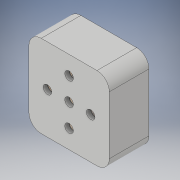
# Autodesk Inventor part: bottom
Saved by Autodesk Inventor 2019 (Build 230136000, 136)
## iProperties
Created: 2019-08-20
Part Number: bottom
Material: Generic
Document SubType Name: Modeling
Designer: assman
Density: 1 g/cm^3
Appearance: Default
Author: assman
## iProperties of the stored document bottom_3DPrint.ipt
Created: 2019-08-20
Part Number: bottom_3DPrint
Material: Generic
Document SubType Name: Modeling
Designer: assman
Density: 1 g/cm^3
Appearance: Default
Author: assman
Autodesk Inventor part; units mm, degrees
ref_plane "YZ Plane" through (0, 0, 0) normal (1, 0, 0) x (0, 1, 0)
ref_plane "XZ Plane" through (0, 0, 0) normal (0, 1, 0) x (-1, 0, 0)
ref_plane "XY Plane" through (0, 0, 0) normal (0, 0, 1) x (1, 0, 0)
ref_plane "Work Plane1" through (0, 0, 0) normal (0, 0, 1) x (-1, 0, 0)
sketch "Sketch1" plane through (0, 0, 0) normal (0, 0, 1) x (-1, 0, 0)
  line L0 (-17.4798, 9.425) -> (-17.4798, -9.425)
  arc A0 (-17.4798, -9.425) -> (-13.4798, -13.425) centre (-13.4798, -9.425) ccw
  line L1 (-13.4798, -13.425) -> (4.6702, -13.425)
  arc A1 (4.6702, -13.425) -> (8.6702, -9.425) centre (4.6702, -9.425) ccw
  line L2 (8.6702, -9.425) -> (8.6702, 9.425)
  arc A2 (8.6702, 9.425) -> (4.6702, 13.425) centre (4.6702, 9.425) ccw
  line L3 (4.6702, 13.425) -> (-0.4048, 13.425)
  line L4 (-0.4048, 13.425) -> (-8.4048, 13.425)
  line L5 (-8.4048, 13.425) -> (-13.4798, 13.425)
  arc A3 (-13.4798, 13.425) -> (-17.4798, 9.425) centre (-13.4798, 9.425) ccw
  constraints: 12 end point, 8 point on circle, 4 centre point
extrude "Extrusion1" add sketch "Sketch1" along normal blind 2
sketch "Sketch2" plane through (0, 0, 0) normal (0, 0, -1) x (-1, 0, 0)
  line L0 (-17.4798, -9.425) -> (-17.4798, 9.425) projected
  arc A0 (-17.4798, -9.425) -> (-13.4798, -13.425) centre (-13.4798, -9.425) ccw projected
  line L1 (4.6702, -13.425) -> (-13.4798, -13.425) projected
  arc A1 (4.6702, -13.425) -> (8.6702, -9.425) centre (4.6702, -9.425) ccw projected
  line L2 (8.6702, 9.425) -> (8.6702, -9.425) projected
  arc A2 (8.6702, 9.425) -> (4.6702, 13.425) centre (4.6702, 9.425) ccw projected
  line L3 (-13.4798, 13.425) -> (4.6702, 13.425) projected
  arc A3 (-13.4798, 13.425) -> (-17.4798, 9.425) centre (-13.4798, 9.425) ccw projected
  arc A4 (7.4702, 9.425) -> (4.6702, 12.225) centre (4.6702, 9.425) ccw
  line L4 (7.4702, 9.425) -> (7.4702, -9.425)
  arc A5 (4.6702, -12.225) -> (7.4702, -9.425) centre (4.6702, -9.425) ccw
  line L5 (4.6702, -12.225) -> (-13.4798, -12.225)
  arc A6 (-16.2798, -9.425) -> (-13.4798, -12.225) centre (-13.4798, -9.425) ccw
  line L6 (-16.2798, -9.425) -> (-16.2798, 9.425)
  arc A7 (-13.4798, 12.225) -> (-16.2798, 9.425) centre (-13.4798, 9.425) ccw
  line L7 (-13.4798, 12.225) -> (4.6702, 12.225)
  point P0 (0, 0)
  dimension "d3" = 1.2
  constraints: 8 end point, 8 point on circle, 4 centre point, 7 other
  measures "d3" distance between parallel lines of L3 L7
ref_plane "Work Plane2" through (2.6548, -1.75, -11.6) normal (0, 0, -1) x (0, 1, 0)
extrude "Extrusion2" add sketch "Sketch2" along normal up to surface (11.6 mm away)
sketch "Sketch3" plane through (0, 0, 0) normal (0, 0, -1) x (-1, 0, 0)
  circle A0 centre (-11.4398, -7.385) radius 1.5 projected
  circle A1 centre (-11.4398, 7.385) radius 1.5 projected
  circle A2 centre (2.6302, 7.385) radius 1.5 projected
  circle A3 centre (2.6302, -7.385) radius 1.5 projected
  circle A4 centre (-11.4398, -7.385) radius 2.5
  circle A5 centre (-11.4398, 7.385) radius 2.5
  circle A6 centre (2.6302, 7.385) radius 2.5
  circle A7 centre (2.6302, -7.385) radius 2.5
  point P0 (0, 0)
  dimension "d8" = 1
  dimension "d9" = 1
  dimension "d10" = 1
  dimension "d11" = 1
  constraints: 4 centre point
  measures "d8" radial gap between concentric circles of A0 A4
  measures "d9" radial gap between concentric circles of A1 A5
  measures "d10" radial gap between concentric circles of A2 A6
  measures "d11" radial gap between concentric circles of A3 A7
ref_plane "Work Plane3" through (-5.6702, -10.425, -4) normal (0, 0, 1) x (1, 0, 0)
extrude "Extrusion3" add sketch "Sketch3" along normal up to surface (4 mm away) contours A0 | A1 | A2 | A3 | A4 | A5 | A6 | A7
sketch "Sketch4" plane through (11.4398, -7.385, -4) normal (0, 0, -1) x (-1, 0, 0)
  point P0 (11.4398, 7.385)
sketch "Sketch5" plane through (11.4398, -7.385, -4) normal (0, 0, -1) x (-1, 0, 0)
  circle A0 centre (0, 0) radius 2.5 projected
  circle A1 centre (0, 14.77) radius 2.5 projected
  circle A2 centre (14.07, 14.77) radius 2.5 projected
  circle A3 centre (14.07, 0) radius 2.5 projected
  point P0 (11.4398, 7.385)
  constraints: 4 coincident
hole "Hole1" at (11.4398, -7.385, -4) at (11.4398, 7.385, -4) at (-2.6302, 7.385, -4) at (-2.6302, -7.385, -4) direction (0, 0, 1) diameter 2.8 depth 4 tip angle 118
fillet "Fillet1" radius 1 4 edges at (13.9398, -7.385, 0) (13.9398, 7.385, 0) (-0.1302, 7.385, 0) (-0.1302, -7.385, 0)
sketch "Sketch6" plane through (0, 0, 0) normal (0, 0, -1) x (-1, 0, 0)
  line L0 (-13.4798, -12.225) -> (4.6702, -12.225) construction
  line L1 (7.4702, -9.425) -> (7.4702, 9.425) construction
  line L2 (-16.2798, 9.425) -> (-16.2798, -9.425) construction
  line L3 (4.6702, 12.225) -> (-13.4798, 12.225) construction
  line L4 (-13.4798, -12.225) -> (4.6702, -12.225) construction
  line L5 (-4.4048, -12.225) -> (-4.4048, 12.225) construction
  line L6 (4.6702, 12.225) -> (-13.4798, 12.225) construction
  line L7 (6.7041, 0) -> (-16.2798, 0) construction
  circle A0 centre (-11.4398, 7.385) radius 1.4 construction
  line L8 (-11.4398, 7.385) -> (-11.4398, -7.385) construction
  circle A1 centre (2.6302, -7.385) radius 1.4 construction
  line L9 (-11.4398, -7.385) -> (2.6302, -7.385) construction
  circle A2 centre (2.6302, 7.385) radius 1.4 construction
  line L10 (2.6302, -7.385) -> (2.6302, 7.385) construction
  line L11 (2.6302, 7.385) -> (-11.4398, 7.385) construction
  circle A3 centre (-11.4398, 0) radius 1.5
  circle A4 centre (-4.4048, -7.385) radius 1.5
  circle A5 centre (2.6302, 0) radius 1.5
  circle A6 centre (-4.4048, 7.385) radius 1.5
  circle A7 centre (-4.4048, 0) radius 1.5
  point P0 (0, 0)
  dimension "d20" = 3
  dimension "d21" = 3
  dimension "d22" = 3
  dimension "d23" = 3
  dimension "d24" = 3
  constraints: 12 end point, 8 midpoint, 5 centre point, 3 perpendicular, 1 point on line, 1 vertical
  measures "d20" diameter of A3
  measures "d21" diameter of A4
  measures "d22" diameter of A5
  measures "d23" diameter of A6
  measures "d24" diameter of A7
hole "Hole2" at (-2.6302, 0, 0) at (11.4398, 0, 0) at (4.4048, 0, 0) at (4.4048, 7.385, 0) at (4.4048, -7.385, 0) direction (0, 0, 1) diameter 2.8 end through all countersink diameter 4 countersink angle 90
fillet "Fillet2" radius 1 8 edges at (-6.6501, 11.4049, 0) (4.4048, 12.225, 0) (15.4597, 11.4049, 0) (16.2798, 0, 0) (15.4597, -11.4049, 0) (4.4048, -12.225, 0) (-6.6501, -11.4049, 0) (-7.4702, 0, 0)
sketch "Sketch7" plane through (-4.6702, -12.225, -11.6) normal (0, 1, 0) x (1, 0, 0)
  line L0 (4.075, -0.84) -> (4.075, -7.04)
  line L1 (4.075, -7.04) -> (14.075, -7.04)
  line L2 (14.075, -7.04) -> (14.075, -0.84)
  line L3 (14.075, -0.84) -> (4.075, -0.84)
  point P0 (4.6702, -11.6)
  constraints: 8 end point
extrude "Extrusion4" cut sketch "Sketch7" against normal blind 2
sketch "Sketch8" plane through (-0.5952, -12.225, -10.76) normal (0, 0, 1) x (1, 0, 0)
  line L0 (10, -1.2) -> (0, -1.2) projected
  line L1 (10, 0) -> (10, -1.2) projected
  line L2 (0, 0) -> (10, 0) projected
  line L3 (0, 0) -> (0, -1.2) projected
  point P0 (0.5952, 12.225)
extrude "Extrusion5" cut sketch "Sketch8" against normal blind 2
fillet "Fillet3" radius 1 2 edges at (9.4048, -12.825, -4.56) (-0.5952, -12.825, -4.56)
sketch "Sketch9" plane through (13.4798, 13.425, -11.6) normal (0, 0, -1) x (-1, 0, 0)
  point P0 (13.4798, -13.425)
sketch "Sketch10" plane through (13.4798, 13.425, -11.6) normal (0, 0, -1) x (-1, 0, 0)
  line L0 (14.075, -25.65) -> (14.075, -26.85) projected
  line L1 (18.15, -26.85) -> (14.075, -26.85) projected
  arc A0 (18.15, -26.85) -> (22.15, -22.85) centre (18.15, -22.85) ccw projected
  line L2 (22.15, -4) -> (22.15, -22.85) projected
  arc A1 (22.15, -4) -> (18.15, 0) centre (18.15, -4) ccw projected
  line L3 (0, 0) -> (18.15, 0) projected
  arc A2 (0, 0) -> (-4, -4) centre (0, -4) ccw projected
  line L4 (-4, -22.85) -> (-4, -4) projected
  arc A3 (-4, -22.85) -> (0, -26.85) centre (0, -22.85) ccw projected
  line L5 (4.075, -26.85) -> (0, -26.85) projected
  line L6 (4.075, -26.85) -> (4.075, -25.65) projected
  line L7 (0, -25.65) -> (4.075, -25.65) projected
  arc A4 (-2.8, -22.85) -> (0, -25.65) centre (0, -22.85) ccw projected
  line L8 (-2.8, -4) -> (-2.8, -22.85) projected
  arc A5 (0, -1.2) -> (-2.8, -4) centre (0, -4) ccw projected
  line L9 (18.15, -1.2) -> (0, -1.2) projected
  arc A6 (20.95, -4) -> (18.15, -1.2) centre (18.15, -4) ccw projected
  line L10 (20.95, -22.85) -> (20.95, -4) projected
  arc A7 (18.15, -25.65) -> (20.95, -22.85) centre (18.15, -22.85) ccw projected
  line L11 (14.075, -25.65) -> (18.15, -25.65) projected
  point P0 (13.4798, -13.425)
ref_plane "Work Plane4" through (-0.0502, -4.455, -10.9) normal (0, 0, -1) x (0, 1, 0)
extrude "Extrusion6" cut sketch "Sketch10" against normal up to surface (0.7 mm away)
body "Solid1"
